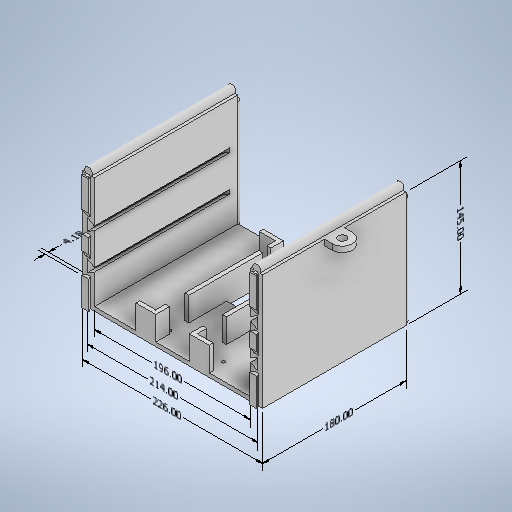
# Autodesk Inventor part: Base
Saved by Autodesk Inventor 2025.1 (Build 291241000, 241)
## iProperties
Created: 2025-11-19
Part Number: Base
Material: Genérico
Document SubType Name: Modeling
Designer: Diego
Density: 1 g/cm^3
Appearance: Valor por defecto
Author: Diego
Autodesk Inventor part; units mm, degrees
ref_plane "YZ Plane" through (0, 0, 0) normal (1, 0, 0) x (0, 1, 0)
ref_plane "XZ Plane" through (0, 0, 0) normal (0, 1, 0) x (-1, 0, 0)
ref_plane "XY Plane" through (0, 0, 0) normal (0, 0, 1) x (1, 0, 0)
sketch "Boceto2" plane through (0, 0, 0) normal (0, 1, 0) x (-1, 0, 0)
  line L0 (-98, 90) -> (98, 90)
  line L1 (98, 90) -> (98, -90)
  line L2 (98, -90) -> (-98, -90)
  line L3 (-98, -90) -> (-98, 90)
  line L4 (-98, 90) -> (98, -90) construction
  line L5 (98, 90) -> (-98, -90) construction
  line L6 (0, -120.4592) -> (0, 245.0518) construction
  line L7 (141.8909, 0) -> (-193.3572, 0) construction
  circle A0 centre (24.5, -69) radius 2
  circle A1 centre (-24.5, -69) radius 2
  line L8 (106.6524, -69) -> (-120.4554, -69) construction
  circle A2 centre (43, -69) radius 2
  circle A3 centre (-43, -69) radius 2
  line L9 (127.2452, 51) -> (-131.3405, 51) construction
  circle A4 centre (21.5, 51) radius 2
  circle A5 centre (-21.5, 51) radius 2
  line L10 (127.2452, 41) -> (-220.4146, 41) construction
  circle A6 centre (43, 41) radius 2
  circle A7 centre (-43, 41) radius 2
  line L11 (-21, 44) -> (21, 44)
  line L12 (21, 44) -> (21, -1)
  line L13 (21, -1) -> (-21, -1)
  line L14 (-21, -1) -> (-21, 44)
  line L15 (-21, 44) -> (21, -1) construction
  line L16 (21, 44) -> (-21, -1) construction
  point P0 (0, 0)
  point P1 (0, 21.5)
  dimension "d0" = 196
  dimension "d1" = 180
  dimension "d2" = 4
  dimension "d3" = 4
  dimension "d4" = 21
  dimension "d5" = 49
  dimension "d6" = 4
  dimension "d7" = 4
  dimension "d8" = 86
  dimension "d10" = 4
  dimension "d11" = 4
  dimension "d12" = 43
  dimension "d13" = 141
  dimension "d14" = 10
  dimension "d15" = 4
  dimension "d16" = 4
  dimension "d17" = 86
  dimension "d18" = 42
  dimension "d19" = 45
  dimension "d20" = 89
  constraints: 34 end point, 9 point on line, 8 centre point, 7 horizontal, 4 midpoint, 4 parallel, 4 symmetric about line, 2 perpendicular, 2 vertical
  measures "d0" distance of L1.end L2.end
  measures "d1" distance of L2.end L0.start
  measures "d2" diameter of A0
  measures "d3" diameter of A1
  measures "d4" distance between parallel lines of L2 L8
  measures "d5" distance of A1.centre A0.centre
  measures "d6" diameter of A2
  measures "d7" diameter of A3
  measures "d8" distance of A3.centre A2.centre
  measures "d10" diameter of A4
  measures "d11" diameter of A5
  measures "d12" distance of A5.centre A4.centre
  measures "d13" distance between parallel lines of L2 L9
  measures "d14" distance between parallel lines of L10 L9
  measures "d15" diameter of A6
  measures "d16" diameter of A7
  measures "d17" distance of A7.centre A6.centre
  measures "d18" distance of L12.end L13.end
  measures "d19" distance of L13.end L11.start
  measures "d20" distance between parallel lines of L2 L13
extrude "Extrusión1" add sketch "Boceto2" along normal blind 5
sketch "Boceto4" plane through (0, 0, 0) normal (0, 1, 0) x (-1, 0, 0)
  line L0 (-98, -90) -> (98, -90) projected
  line L1 (98, -90) -> (98, 90) projected
  line L2 (98, 90) -> (-98, 90) projected
  line L3 (-98, 90) -> (-98, -90) projected
  line L4 (113, -90) -> (113, 90)
  line L5 (-113, -90) -> (-113, 90)
  line L6 (203.0929, 0) -> (-180.6061, 0) construction
  line L7 (113, -90) -> (98, -90)
  line L8 (98, -90) -> (98, 90)
  line L9 (113, 90) -> (98, 90)
  line L10 (-98, -90) -> (-113, -90)
  line L11 (-113, 90) -> (-98, 90)
  line L12 (-98, 90) -> (-98, -90)
  point P0 (0, 0)
  point P1 (113, 0)
  point P2 (-113, 0)
  dimension "d25" = 15
  dimension "d26" = 15
  constraints: 18 end point, 4 parallel, 3 horizontal, 2 collinear, 2 midpoint, 2 point on line, 2 vertical, 1 perpendicular
  measures "d25" distance between parallel lines of L1 L4
  measures "d26" distance between parallel lines of L5 L3
extrude "Extrusión2" add sketch "Boceto4" along normal blind 145 contours L10 L5 L11 L3 | L1 L9 L4 L7
sketch "Boceto5" plane through (0, 5, 0) normal (0, 1, 0) x (1, 0, 0)
  line L0 (-113, -90) -> (-113, 90) projected
  line L1 (-113, 90) -> (-98, 90) projected
  line L2 (-98, 90) -> (-98, -90) projected
  line L3 (98, -90) -> (-98, -90) projected
  line L4 (98, -90) -> (98, 90) projected
  line L5 (98, 90) -> (113, 90) projected
  line L6 (113, 90) -> (113, -90) projected
  line L7 (113, -90) -> (98, -90) projected
  line L8 (-98, -90) -> (-113, -90) projected
  line L9 (-98, 90) -> (98, 90) projected
  line L10 (21, -44) -> (21, 1) projected
  line L11 (21, 1) -> (-21, 1) projected
  line L12 (-21, 1) -> (-21, -44) projected
  line L13 (-21, -44) -> (21, -44) projected
  circle A0 centre (-24.5, 69) radius 2 projected
  circle A1 centre (24.5, 69) radius 2 projected
  circle A2 centre (-43, 69) radius 2 projected
  circle A3 centre (43, 69) radius 2 projected
  circle A4 centre (-21.5, -51) radius 2 projected
  circle A5 centre (21.5, -51) radius 2 projected
  circle A6 centre (-43, -41) radius 2 projected
  circle A7 centre (43, -41) radius 2 projected
  line L14 (98, 90) -> (-98, 90) projected
  line L15 (21, -44) -> (26, -44)
  line L16 (26, 48.4181) -> (21, 48.4181)
  line L17 (158.8769, 0) -> (-159.3491, 0) construction
  line L18 (0, -90) -> (0, 90) construction
  line L19 (-21, -44) -> (-21, 1)
  line L20 (26, 85) -> (46, 85)
  line L21 (21, 90) -> (46, 90)
  line L22 (46, 85) -> (46, 90)
  line L23 (26, 85) -> (26, 73)
  line L24 (26, 73) -> (21, 73)
  line L25 (21, -44) -> (21, 48.4181)
  line L26 (21, 73) -> (21, 90)
  line L27 (26, -44) -> (26, 48.4181)
  line L28 (21, -54.5) -> (21, -70)
  line L29 (21, -70) -> (46, -70)
  line L30 (46, -70) -> (46, -65)
  line L31 (46, -65) -> (26, -65)
  line L32 (26, -65) -> (26, -54.5)
  line L33 (26, -54.5) -> (21, -54.5)
  line L34 (21, 1) -> (21, -44) projected
  line L35 (98, 90) -> (-98, 90) projected
  line L36 (-98, 90) -> (-98, -90) projected
  line L37 (-98, -90) -> (98, -90) projected
  line L38 (98, -90) -> (98, 90) projected
  circle A8 centre (43, -41) radius 2 projected
  circle A9 centre (-43, -41) radius 2 projected
  circle A10 centre (21.5, -51) radius 2 projected
  circle A11 centre (-21.5, -51) radius 2 projected
  circle A12 centre (43, 69) radius 2 projected
  circle A13 centre (-43, 69) radius 2 projected
  circle A14 centre (24.5, 69) radius 2 projected
  circle A15 centre (-24.5, 69) radius 2 projected
  line L39 (21, -44) -> (-21, -44) projected
  line L40 (-21, -44) -> (-21, 1) projected
  line L41 (-21, 1) -> (21, 1) projected
  line L42 (21, 1) -> (21, -44) projected
  line L43 (-21, -54.5) -> (-21, -70)
  line L44 (-21, -70) -> (-46, -70)
  line L45 (-46, -70) -> (-46, -65)
  line L46 (-46, -65) -> (-26, -65)
  line L47 (-26, -65) -> (-26, -54.5)
  line L48 (-26, -54.5) -> (-21, -54.5)
  line L49 (-26, 85) -> (-46, 85)
  line L50 (-21, 90) -> (-46, 90)
  line L51 (-46, 85) -> (-46, 90)
  line L52 (-26, 85) -> (-26, 73)
  line L53 (-26, 73) -> (-21, 73)
  line L54 (-21, 73) -> (-21, 90)
  line L55 (-21, -44) -> (-21, 1)
  line L56 (-21, -44) -> (-26, -44)
  line L57 (-26, 48.4181) -> (-21, 48.4181)
  line L58 (-21, -44) -> (-21, 48.4181)
  line L59 (-26, -44) -> (-26, 48.4181)
  line L60 (-21, 1) -> (-21, -44)
  line L61 (-21, 1) -> (-21, -44)
  point P0 (0, 0)
  dimension "d32" = 20
  dimension "d34" = 5
  dimension "d35" = 5
  dimension "d39" = 5
  dimension "d40" = 25
  dimension "d41" = 5
  dimension "d42" = 20
  dimension "d43" = 150
  dimension "d44" = 15.5
  dimension "d45" = 17
  constraints: 76 end point, 19 symmetric about line, 11 perpendicular, 4 horizontal, 3 parallel, 3 vertical, 2 collinear, 2 point on line, 1 midpoint
  measures "d32" distance of L20.start L20.end
  measures "d34" distance between parallel lines of L9 L20
  measures "d35" distance between parallel lines of L26 L23
  measures "d39" distance between parallel lines of L25 L27
  measures "d40" distance of L28.end L29.end
  measures "d41" distance of L29.end L30.end
  measures "d42" distance of L30.end L31.end
  measures "d43" distance between parallel lines of L31 L20
  measures "d44" distance between parallel lines of L29 L33
  measures "d45" distance between parallel lines of L9 L24
extrude "Extrusión3" add sketch "Boceto5" along normal blind 30 contours L9 L54 L53 L52 L49 L51 | L22 L20 L23 L24 L26 L9 | L10 L25 L16 L27 L15 | L56 L59 L57 L58 L12 | L33 L32 L31 L30 L29 L28 | L43 L44 L45 L46 L47 L48
sketch "Boceto6" plane through (113, 0, -90) normal (0, 0, -1) x (-1, 0, 0)
  line L0 (226, 145) -> (226, 0) projected
  line L1 (226, 0) -> (0, 0) projected
  line L2 (0, 0) -> (0, 145) projected
  line L3 (0, 145) -> (15, 145) projected
  line L4 (15, 145) -> (15, 5) projected
  line L5 (15, 5) -> (67, 5) projected
  line L6 (67, 5) -> (67, 35) projected
  line L7 (67, 35) -> (92, 35) projected
  line L8 (92, 35) -> (92, 5) projected
  line L9 (92, 5) -> (134, 5) projected
  line L10 (134, 5) -> (134, 35) projected
  line L11 (134, 35) -> (159, 35) projected
  line L12 (159, 35) -> (159, 5) projected
  line L13 (159, 5) -> (211, 5) projected
  line L14 (211, 5) -> (211, 145) projected
  line L15 (211, 145) -> (226, 145) projected
  line L16 (226, 45) -> (-12.5381, 45) construction
  line L17 (15, 50) -> (15, 47.5)
  line L18 (15, 47.5) -> (6, 52.6962)
  line L19 (6, 52.6962) -> (6, 37.3038)
  line L20 (6, 37.3038) -> (15, 42.5)
  line L21 (15, 40) -> (15, 42.5)
  line L22 (15, 47.5) -> (15, 50)
  line L23 (15, 5) -> (15, 145) projected
  line L24 (15, 47.5) -> (24.0333, 47.5) construction
  line L25 (15, 42.5) -> (24.4759, 42.5) construction
  line L26 (113, 0) -> (113, 106.3202) construction
  line L27 (15, 50) -> (15, 47.5) construction
  line L28 (15, 42.5) -> (15, 40) construction
  line L29 (15, 50) -> (15, 47.5) construction
  line L30 (15, 40) -> (15, 42.5) construction
  line L31 (211, 50) -> (211, 47.5)
  line L32 (211, 47.5) -> (220, 52.6962)
  line L33 (220, 52.6962) -> (220, 37.3038)
  line L34 (220, 37.3038) -> (211, 42.5)
  line L35 (211, 42.5) -> (211, 42.5)
  line L36 (211, 47.5) -> (211, 50)
  line L37 (211, 50) -> (211, 47.5) construction
  line L38 (211, 42.5) -> (211, 42.5) construction
  line L39 (211, 50) -> (211, 47.5) construction
  line L40 (211, 42.5) -> (211, 42.5) construction
  line L41 (15, 50) -> (15, 47.5)
  line L42 (15, 42.5) -> (15, 40)
  line L43 (211, 50) -> (211, 47.5)
  line L44 (211, 45) -> (211, 42.5)
  line L45 (211, 50) -> (211, 45)
  line L46 (211, 42.5) -> (211, 42.5)
  line L47 (15, 40) -> (211, 40) construction
  line L48 (211, 50) -> (15, 50) construction
  line L49 (15, 95) -> (15, 92.5)
  line L50 (15, 92.5) -> (6, 97.6962)
  line L51 (6, 97.6962) -> (6, 82.3038)
  line L52 (6, 82.3038) -> (15, 87.5)
  line L53 (15, 85) -> (15, 87.5)
  line L54 (15, 92.5) -> (15, 95)
  line L55 (15, 92.5) -> (24.0333, 92.5) construction
  line L56 (15, 87.5) -> (24.4759, 87.5) construction
  line L57 (15, 95) -> (15, 92.5) construction
  line L58 (15, 87.5) -> (15, 85) construction
  line L59 (15, 95) -> (15, 92.5) construction
  line L60 (15, 85) -> (15, 87.5) construction
  line L61 (15, 95) -> (15, 92.5)
  line L62 (15, 85) -> (211, 85) construction
  line L63 (211, 95) -> (15, 95) construction
  line L64 (15, 92.5) -> (15, 87.5)
  line L65 (211, 95) -> (211, 92.5)
  line L66 (211, 92.5) -> (211, 95)
  line L67 (211, 95) -> (211, 92.5)
  line L68 (211, 95) -> (211, 92.5) construction
  line L69 (220, 82.3038) -> (211, 87.5)
  line L70 (220, 97.6962) -> (220, 82.3038)
  line L71 (211, 92.5) -> (220, 97.6962)
  line L72 (211, 95) -> (211, 92.5) construction
  line L73 (211, 87.5) -> (211, 85) construction
  line L74 (211, 85) -> (211, 87.5) construction
  line L75 (211, 85) -> (211, 87.5)
  line L76 (211, 92.5) -> (211, 87.5)
  point P0 (6, 45)
  point P1 (220, 45)
  point P2 (6, 90)
  point P3 (19.5166, 92.5)
  point P4 (10.5, 95.0981)
  point P5 (211, 85)
  point P6 (211, 95)
  point P7 (220, 90)
  point P8 (215.5, 95.0981)
  point P9 (15, 92.5)
  dimension "d52" = 60
  dimension "d53" = 2.5
  dimension "d57" = 9
  dimension "d65" = 10
  dimension "d66" = 60
  dimension "d67" = 10
  dimension "d68" = 35
  dimension "d69" = 35
  dimension "d70" = 2.5
  dimension "d71" = 2.5
  constraints: 120 end point, 15 symmetric about line, 12 collinear, 10 horizontal, 9 point on line, 5 midpoint, 5 vertical, 2 parallel, 1 perpendicular, 4 other
  measures "d52" angle of L18 L19
  measures "d53" distance between parallel lines of L16 L24
  measures "d57" distance between parallel lines of L4 L19
  measures "d65" distance between parallel lines of L47 L48
  measures "d66" angle of L50 L51
  measures "d67" distance between parallel lines of L62 L63
  measures "d68" distance between parallel lines of L5 L47
  measures "d69" distance between parallel lines of L48 L62
  measures "d70" distance from line of L63 point (19.517, 92.5)
  measures "d71" distance between parallel lines of L62 L56
extrude "Extrusión4" cut sketch "Boceto6" against normal blind 170 contours L71 L70 L69 L14 | L4 L52 L51 L50 | L32 L33 L34 L14 | L4 L20 L19 L18
sketch "Boceto7" plane through (0, 145, 0) normal (0, 1, 0) x (1, 0, 0)
  line L0 (98, -90) -> (113, -90) projected
  line L1 (-113, -90) -> (-98, -90) projected
  line L2 (105.5, -90) -> (105.5, -56.437) construction
  line L3 (105.5, -90) -> (105.5, -123.7842) construction
  line L4 (0, 0) -> (0, -202.84) construction
  arc A0 (101.5942, -90) -> (109.4058, -90) centre (105.5, -93) ccw
  arc A1 (-109.4058, -90) -> (-101.5942, -90) centre (-105.5, -93) ccw
  point P0 (-105.5, -90)
  point P1 (-101.5942, -90)
  point P2 (-109.4058, -90)
  dimension "d58" = 3
  dimension "d59" = 9.85
  constraints: 6 end point, 4 point on circle, 4 symmetric about line, 3 point on line, 3 vertical, 2 centre point, 1 midpoint, 1 other
  measures "d58" distance from line of L0 A0.centre
  measures "d59" diameter of A0
extrude "Extrusión5" add sketch "Boceto7" against normal blind 145
sketch "Boceto8" plane through (0, 145, 0) normal (0, 1, 0) x (1, 0, 0)
  line L0 (-113, -90) -> (113, -90) projected
  line L1 (113, -90) -> (-113, -90)
  line L2 (-113, -90) -> (-113, -105)
  line L3 (-113, -105) -> (113, -105)
  line L4 (113, -105) -> (113, -90)
  line L5 (-113, 90) -> (-113, -90) projected
  point P0 (0, 0)
  point P1 (109.4058, -90)
  point P2 (107.3028, -90)
  dimension "d62" = 15
  constraints: 8 end point, 2 parallel, 1 collinear, 1 horizontal, 1 perpendicular
  measures "d62" distance between parallel lines of L1 L3
extrude "Extrusión6" cut sketch "Boceto8" against normal blind 10
sketch "Boceto9" plane through (113, 0, -90) normal (0, 0, -1) x (-1, 0, 0)
  line L0 (0, 145) -> (15, 145) projected
  line L1 (7.5, 145) -> (7.5, 175.346) construction
  arc A0 (11.4058, 145) -> (3.5942, 145) centre (7.5, 148) ccw
  line L2 (113, 0) -> (113, 199.4822) construction
  arc A1 (222.4058, 145) -> (214.5942, 145) centre (218.5, 148) ccw
  line L3 (211, 145) -> (226, 145) projected
  dimension "d87" = 9.85
  dimension "d88" = 3
  constraints: 4 end point, 4 point on circle, 3 point on line, 3 symmetric about line, 2 centre point, 2 vertical, 1 midpoint, 1 other
  measures "d87" diameter of A0
  measures "d88" distance from line of L0 A0.centre
extrude "Extrusión7" add sketch "Boceto9" against normal blind 180
sketch "Boceto10" plane through (0, 145, 0) normal (0, 1, 0) x (1, 0, 0)
  line L0 (-113, 90) -> (-113, -90) construction
  line L1 (-113, 0) -> (-204.3255, 0) construction
  line L2 (-113, -12.5) -> (-123, -12.5)
  line L3 (-123, -12.5) -> (-123, 12.5)
  line L4 (-123, 12.5) -> (-113, 12.5)
  line L5 (-113, 12.5) -> (-113, -12.5)
  circle A0 centre (-123, 0) radius 5
  arc A1 (-123, 12.5) -> (-123, -12.5) centre (-123, 0) ccw
  point P0 (0, 0)
  dimension "d91" = 10
  dimension "d92" = 25
  dimension "d93" = 10
  constraints: 10 end point, 2 centre point, 2 horizontal, 2 midpoint, 2 parallel, 2 point on circle, 1 coincident, 1 perpendicular, 1 point on line, 1 other
  measures "d91" distance of L3.end L4.end
  measures "d92" distance of L3.end L2.end
  measures "d93" diameter of A0
extrude "Extrusión8" add sketch "Boceto10" against normal blind 7 contours L2 L3 A0 L4 L5 | A1 L3 A0
sketch "Boceto12" plane through (0, 145, 0) normal (0, 1, 0) x (1, 0, 0)
  line L0 (113, 90) -> (-113, 90) projected
  line L1 (-113, 90) -> (-107, 90)
  line L2 (0, 90) -> (0, 142.1234) construction
  line L3 (-100.575, 90) -> (-110.425, 90) projected
  line L4 (-109.4058, 90) -> (-113, 90) projected
  line L5 (-110.425, 90) -> (-110.425, -90) projected
  line L6 (-110.425, 90) -> (-110.425, -90) projected
  line L7 (-110.425, 90) -> (-107, 90)
  line L8 (-107, 90) -> (-110.425, 90)
  line L9 (-113, 90) -> (-113, 12.5) projected
  line L10 (-113, 90) -> (-107, 90) construction
  line L11 (-110.425, 90) -> (-107, 90)
  line L12 (-110.425, 90) -> (-107, 90)
  line L13 (-113, 90) -> (113, 90)
  line L14 (-109.4058, 90) -> (-101.5942, 90) projected
  line L15 (-109.4058, -90) -> (-109.4058, 90) projected
  line L16 (-101.5942, -90) -> (-109.4058, -90) projected
  line L17 (-101.5942, 90) -> (-101.5942, -90) projected
  line L18 (-101.5942, 90) -> (-109.4058, 90) construction
  line L19 (-105.5, 90) -> (-105.5, 105.6895) construction
  line L20 (-103, 90) -> (-108, 90) construction
  line L21 (-108, 90) -> (-108, 94.3301) construction
  line L22 (-108, 94.3301) -> (-103, 94.3301) construction
  line L23 (-103, 94.3301) -> (-103, 90) construction
  line L24 (-103, 90) -> (-100.5, 94.3301) construction
  line L25 (-100.5, 94.3301) -> (-110.5, 94.3301) construction
  line L26 (-110.5, 94.3301) -> (-108, 90) construction
  line L27 (-103, 90) -> (-108, 90)
  line L28 (-103, 90) -> (-108, 90)
  line L29 (-103.1732, 90) -> (-100.7598, 94.1801)
  line L30 (-100.7598, 94.1801) -> (-110.2402, 94.1801)
  line L31 (-110.2402, 94.1801) -> (-107.8268, 90)
  line L32 (103.1732, 90) -> (100.7598, 94.1801)
  line L33 (100.7598, 94.1801) -> (110.2402, 94.1801)
  line L34 (110.2402, 94.1801) -> (107.8268, 90)
  point P0 (0, 0)
  point P1 (-105.5, 90)
  dimension "d113" = 5
  dimension "d115" = 60
  dimension "d116" = 10
  dimension "d117" = 0.15
  dimension "d123" = 7.5
  constraints: 50 end point, 6 horizontal, 6 symmetric about line, 4 point on line, 3 collinear, 3 parallel, 2 midpoint, 2 vertical, 1 perpendicular, 6 other
  measures "d113" distance of L21.end L22.end
  measures "d115" angle of L25 L24
  measures "d116" distance of L24.end L25.end
  measures "d117" distance between parallel lines of L24 L29
  measures "d123" distance of L1.start point (-105.5, 90)
extrude "Extrusión11" add sketch "Boceto12" against normal blind 145 contours L0 L32 L33 L34 | L0 L31 L30 L29
sketch "Boceto14" plane through (98, 47.5, -90) normal (0, 0, -1) x (-1, 0, 0)
  line L0 (-9, 50.1962) -> (0, 45) projected
  line L1 (-9, 34.8038) -> (-9, 50.1962) projected
  line L2 (0, 40) -> (-9, 34.8038) projected
  line L3 (-15, -47.5) -> (-15, 97.5) projected
  line L4 (205, 50.1962) -> (205, 34.8038) projected
  line L5 (211, -47.5) -> (211, 97.5) projected
  line L6 (205, 5.1962) -> (205, -10.1962) projected
  line L7 (-9, -10.1962) -> (-9, 5.1962) projected
  line L8 (-9, 5.1962) -> (0, 0) projected
  line L9 (0, -5) -> (-9, -10.1962) projected
  line L10 (205, -10.1962) -> (196, -5) projected
  line L11 (196, 0) -> (205, 5.1962) projected
  line L12 (205, 34.8038) -> (196, 40) projected
  line L13 (196, 45) -> (205, 50.1962) projected
  line L14 (-15, 52.1962) -> (211, 52.1962)
  line L15 (211, 52.1962) -> (211, 32.8038)
  line L16 (211, 32.8038) -> (-15, 32.8038)
  line L17 (-15, 32.8038) -> (-15, 52.1962)
  line L18 (-9, 42.5) -> (205, 42.5) construction
  line L19 (0, 40) -> (0, 0) construction
  line L20 (0, 20) -> (196, 20) construction
  line L21 (196, -42.5) -> (196, 97.5) construction
  line L22 (-15, -12.1962) -> (211, -12.1962)
  line L23 (211, 7.1962) -> (-15, 7.1962)
  line L24 (-9, -2.5) -> (205, -2.5) construction
  point P0 (98, -47.5)
  point P1 (-15, 7.1962)
  point P2 (-15, -12.1962)
  point P3 (211, -12.1962)
  point P4 (-15, 32.8038)
  point P5 (211, 52.1962)
  dimension "d120" = 2
  constraints: 20 end point, 6 symmetric about line, 3 midpoint, 3 point on line, 2 parallel, 2 perpendicular, 1 horizontal, 1 vertical, 1 other
  measures "d120" distance from line of L14 L0.start
extrude "Extrusión12" cut sketch "Boceto14" along normal blind 10 contours L3 L23 L5 L22 | L3 L14 L5 L16
chamfer "Chaflán1" distance 4.18 angle 60 1 edges at (105.5, 99.6962, -94.1801) measured on face at (104.7244, 99.6962, -92.7868)
chamfer "Chaflán2" distance 4.18 angle 60 1 edges at (105.5, 54.6962, -94.1801) measured on face at (104.7244, 54.6962, -92.7868)
chamfer "Chaflán3" distance 4.18 angle 60 1 edges at (-105.5, 54.6962, -94.1801) measured on face at (-104.7244, 54.6962, -92.7868)
chamfer "Chaflán4" distance 4.18 angle 60 1 edges at (-105.5, 99.6962, -94.1801) measured on face at (-104.7244, 99.6962, -92.7868)
chamfer "Chaflán5" distance 1 angle 45 6 edges at (101.9665, 145, -92.0901) (105.5, 145, -94.1801) (109.0335, 145, -92.0901) (-109.0335, 145, -92.0901) (-105.5, 145, -94.1801) (-101.9665, 145, -92.0901)
fillet "Empalme1" radius 0.2 12 edges at (100.7598, 125.4681, -94.1801) (110.2402, 125.4681, -94.1801) (110.2402, 71.12, -94.1801) (100.7598, 71.12, -94.1801) (110.2402, 17.6519, -94.1801) (100.7598, 17.6519, -94.1801) (-110.2402, 17.6519, -94.1801) (-100.7598, 17.6519, -94.1801) (-110.2402, 71.12, -94.1801) (-100.7598, 71.12, -94.1801) (-110.2402, 125.4681, -94.1801) (-100.7598, 125.4681, -94.1801)
equation "\"d0\" = W_base"
equation "\"d1\" = L_base"
equation "\"d21\" = T_base"
equation "\"d25\" = T_pared"
equation "\"d26\" = T_pared"
equation "\"d27\" = H_pared"
equation "\"d53\" = 0.25 * T_suelo"
equation "\"d60\" = H_pared"
equation "\"d89\" = L_base"
equation "\"d118\" = H_pared"
equation "\"W_base\" = 196"
equation "\"L_base\" = 180"
equation "\"T_base\" = 5"
equation "\"T_pared\" = 15"
equation "\"H_pared\" = 145"
equation "\"T_suelo\" = 10"
